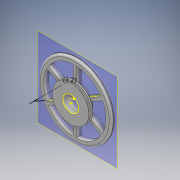
# Autodesk Inventor part: 뒷바퀴
Saved by Autodesk Inventor 2018 (Build 220112000, 112)
## iProperties
Created: 2019-11-05
Part Number: 뒷바퀴
Material: 일반
Document SubType Name: Modeling
Designer: LeeYounSeo
Density: 1 g/cm^3
Appearance: 기본값
Author: LeeYounSeo
Autodesk Inventor part; units mm, degrees
ref_plane "YZ Plane" through (0, 0, 0) normal (1, 0, 0) x (0, 1, 0)
ref_plane "XZ Plane" through (0, 0, 0) normal (0, 1, 0) x (-1, 0, 0)
ref_plane "XY Plane" through (0, 0, 0) normal (0, 0, 1) x (1, 0, 0)
sketch "스케치1" plane through (0, 0, 0) normal (0, 1, 0) x (-1, 0, 0)
  circle A0 centre (0, 0) radius 35
  circle A1 centre (0, 0) radius 7.5
  circle A2 centre (0, 0) radius 12.5
  circle A3 centre (0, 0) radius 30
  dimension "d0" = 70
  dimension "d1" = 15
  dimension "d2" = 25
  dimension "d3" = 60
  constraints: 4 centre point, 4 coincident
  measures "d0" diameter of A0
  measures "d1" diameter of A1
  measures "d2" diameter of A2
  measures "d3" diameter of A3
extrude "돌출1" add sketch "스케치1" along normal blind 5
sketch "스케치2" plane through (0, 0, 0) normal (0, -1, 0) x (1, 0, 0)
  line L0 (-10.8253, 6.25) -> (-25.9808, 15)
  circle A0 centre (0, 0) radius 30 projected
  circle A1 centre (0, 0) radius 7.5 projected
  circle A2 centre (0, 0) radius 7.5 projected
  circle A3 centre (0, 0) radius 12.5 projected
  circle A4 centre (0, 0) radius 12.5 projected
  line L1 (0, 12.5) -> (0, 30)
  line L2 (10.8253, 6.25) -> (25.9808, 15)
  line L3 (10.8253, -6.25) -> (25.9808, -15)
  line L4 (0, -12.5) -> (0, -30)
  line L5 (-10.8253, -6.25) -> (-25.9808, -15)
  line L6 (-1.5, 34.9678) -> (1.5, 34.9678)
  line L7 (1.5, 34.9678) -> (1.5, 12.4097)
  line L8 (1.5, 12.4097) -> (-1.5, 12.4097)
  line L9 (-1.5, 12.4097) -> (-1.5, 34.9678)
  circle A5 centre (0, 0) radius 35 projected
  dimension "d10" = 3
  dimension "d11" = 1.5
  constraints: 20 end point, 14 point on circle, 3 equal length, 1 horizontal, 1 perpendicular, 1 vertical alignment, 2 other
  measures "d10" distance between parallel lines of L7 L9
  measures "d11" distance between parallel lines of L1 L7
extrude "돌출2" add sketch "스케치2" against normal blind 5 contours L9 A0 L1 A3 | L9 L6 L7 A0 | L1 A0 L7 A3
pattern_circular "원형 패턴1" count 6 over 360 about axis through (0, 0, 0) along (0, 1, 0) of "돌출2"
fillet "모깎기1" radius 1.9 2 edges at (35, 0, 0) (35, 5, 0)
sketch "스케치3" plane through (-26.6983, 0, -13.6822) normal (-0.5, 0, 0.866) x (0.866, 0, 0.5)
  line L0 (64.9625, 3.1) -> (-5.0375, 3.1) projected
  line L1 (-5.0375, 1.9) -> (64.9625, 1.9) projected
  point P0 (29.9625, 0)
  dimension "d18" = 1.2
  measures "d18" distance between parallel lines of L0 L1
ref_plane "작업 평면1" through (0, 2.5, 0) normal (0, 1, 0) x (1, 0, 0)
sketch "스케치4" plane through (0, 2.5, 0) normal (0, 1, 0) x (1, 0, 0)
  circle A0 centre (0, 0) radius 35 projected
  circle A1 centre (0, 0) radius 34.4
  dimension "d19" = 0.6
  constraints: 1 centre point
  measures "d19" radial gap between concentric circles of A0 A1
extrude "돌출3" cut sketch "스케치4" along normal mid plane 1.2
sketch "스케치5" plane through (0, 5, 0) normal (0, 1, 0) x (1, 0, 0)
  point P0 (0, 0)
sketch "스케치6" plane through (0, 0, 0) normal (0, -1, 0) x (1, 0, 0)
  arc A0 (9.9971, 7.5039) -> (1.5, 12.4097) centre (0, 0) ccw projected
  circle A1 centre (0, 0) radius 12.5
  line L0 (-9.9971, 7.5039) -> (-25.1983, 16.2803) projected
  arc A2 (-1.5, 29.9625) -> (-25.1983, 16.2803) centre (0, 0) ccw projected
  line L1 (-1.5, 29.9625) -> (-1.5, 12.4097) projected
  arc A3 (-1.5, 12.4097) -> (-9.9971, 7.5039) centre (0, 0) ccw projected
  circle A4 centre (0, 0) radius 7.5 projected
  arc A5 (9.9971, 7.5039) -> (1.5, 12.4097) centre (0, 0) ccw projected
  line L2 (1.5, 12.4097) -> (1.5, 29.9625) projected
  arc A6 (25.1983, 16.2803) -> (1.5, 29.9625) centre (0, 0) ccw projected
  line L3 (25.1983, 16.2803) -> (9.9971, 7.5039) projected
  arc A7 (11.4971, -4.9058) -> (11.4971, 4.9058) centre (0, 0) ccw projected
  line L4 (11.4971, 4.9058) -> (26.6983, 13.6822) projected
  arc A8 (26.6983, -13.6822) -> (26.6983, 13.6822) centre (0, 0) ccw projected
  line L5 (26.6983, -13.6822) -> (11.4971, -4.9058) projected
  arc A9 (1.5, -12.4097) -> (9.9971, -7.5039) centre (0, 0) ccw projected
  line L6 (9.9971, -7.5039) -> (25.1983, -16.2803) projected
  arc A10 (1.5, -29.9625) -> (25.1983, -16.2803) centre (0, 0) ccw projected
  line L7 (1.5, -29.9625) -> (1.5, -12.4097) projected
  arc A11 (-9.9971, -7.5039) -> (-1.5, -12.4097) centre (0, 0) ccw projected
  line L8 (-1.5, -12.4097) -> (-1.5, -29.9625) projected
  arc A12 (-25.1983, -16.2803) -> (-1.5, -29.9625) centre (0, 0) ccw projected
  line L9 (-25.1983, -16.2803) -> (-9.9971, -7.5039) projected
  arc A13 (-11.4971, 4.9058) -> (-11.4971, -4.9058) centre (0, 0) ccw projected
  line L10 (-11.4971, -4.9058) -> (-26.6983, -13.6822) projected
  arc A14 (-26.6983, 13.6822) -> (-26.6983, -13.6822) centre (0, 0) ccw projected
  line L11 (-26.6983, 13.6822) -> (-11.4971, 4.9058) projected
  circle A15 centre (0, 0) radius 33.1 projected
  circle A16 centre (0, 0) radius 17.5
  dimension "d22" = 35
  constraints: 2 coincident, 1 centre point, 3 other
  measures "d22" diameter of A16
extrude "돌출4" add sketch "스케치6" along normal blind 1 contours A1 A0 | L3 A16 L4 A1 | A0 L2 A16 L3 | A1 L1 A16 L2 | L4 A16 L5 A1 | A1 L0 A16 L1 | A1 L11 A16 L0 | L5 A16 L6 A1 | A1 L10 A16 L11 | L6 A16 L7 A1 | A1 L9 A16 L10 | L7 A16 L8 A1 | A1 L8 A16 L9
sketch "스케치7" plane through (0, -1, 0) normal (0, -1, 0) x (1, 0, 0)
  circle A0 centre (0, 0) radius 12.5
  circle A1 centre (0, 0) radius 7.5 projected
  circle A2 centre (0, 0) radius 7.5 projected
  circle A3 centre (0, 0) radius 17.5 projected
  dimension "d25" = 25
  constraints: 1 centre point, 1 coincident
  measures "d25" diameter of A0
extrude "돌출5" add sketch "스케치7" along normal blind 3 contours A0
sketch "스케치8" plane through (0, -4, 0) normal (0, -1, 0) x (1, 0, 0)
  circle A0 centre (0, 0) radius 17.5
  circle A1 centre (0, 0) radius 17.5 projected
  circle A2 centre (0, 0) radius 7.5 projected
  circle A3 centre (0, 0) radius 12.5 projected
  dimension "d28" = 35
  constraints: 1 centre point, 1 coincident
  measures "d28" diameter of A0
extrude "돌출6" add sketch "스케치8" against normal blind 1 contours A0
sketch "스케치9" plane through (0, -4, 0) normal (0, -1, 0) x (1, 0, 0)
  circle A0 centre (0, 0) radius 7.5 projected
sketch "스케치10" plane through (0, -3, 0) normal (0, 1, 0) x (-1, 0, 0)
  point P0 (0, 0)
fillet "모깎기2" radius 0.8 2 edges at (-17.5, -3, 0) (-17.5, -1, 0)
